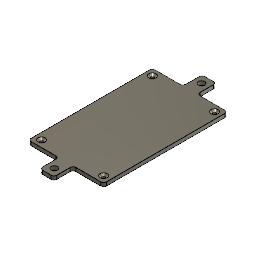
PSU Bracket v1 (Autodesk Fusion 360 design; units mm, degrees)
Autodesk Fusion 360 part; units mm, degrees
sketch "Sketch1" plane through (0, 0, 0) normal (0, 1, 0) x (1, 0, 0)
  line L0 (32.5, 58) -> (-32.5, 58) construction
  line L1 (-32.5, 58) -> (-32.5, -58) construction
  line L2 (-32.5, -58) -> (32.5, -58) construction
  line L3 (32.5, -58) -> (32.5, 58) construction
  line L4 (32.5, 58) -> (-32.5, -58) construction
  line L5 (-32.5, 58) -> (32.5, -58) construction
  circle A0 centre (32.5, 58) radius 1.75
  line L6 (0, 0) -> (0, 14) construction
  line L7 (0, 0) -> (-15, 0) construction
  circle A1 centre (-32.5, 58) radius 1.75
  circle A2 centre (32.5, -58) radius 1.75
  circle A3 centre (-32.5, -58) radius 1.75
  line L8 (39.5, 65) -> (-39.5, 65)
  line L9 (-39.5, 65) -> (-39.5, -65)
  line L10 (-39.5, -65) -> (39.5, -65)
  line L11 (39.5, -65) -> (39.5, 65)
  line L12 (39.5, 65) -> (-39.5, -65) construction
  line L13 (-39.5, 65) -> (39.5, -65) construction
  line L14 (7.5, 85) -> (-7.5, 85)
  line L15 (-7.5, 85) -> (-7.5, 65)
  line L16 (-7.5, 65) -> (7.5, 65)
  line L17 (7.5, 65) -> (7.5, 85)
  line L18 (7.5, 85) -> (-7.5, 65) construction
  line L19 (-7.5, 85) -> (7.5, 65) construction
  circle A4 centre (0, 77) radius 3.25
  line L20 (-7.5, -85) -> (-7.5, -65)
  line L21 (7.5, -85) -> (-7.5, -85)
  line L22 (-7.5, -85) -> (7.5, -65) construction
  circle A5 centre (0, -77) radius 3.25
  line L23 (-7.5, -65) -> (7.5, -65)
  line L24 (7.5, -65) -> (7.5, -85)
  line L25 (7.5, -85) -> (-7.5, -65) construction
  point P0 (0, 75)
  point P1 (0, -75)
  dimension "d1" = 116
  dimension "d2" = 65
  dimension "d3" = 3.5
  dimension "d4" = 7
  dimension "d5" = 7
  dimension "d6" = 20
  dimension "d7" = 15
  dimension "d8" = 6.5
  dimension "d9" = 12
  constraint perpendicular L0 L1
  constraint parallel L0 L2
  constraint parallel L1 L3
  constraint horizontal L0
  constraint coincident L4 L6.start
  constraint coincident L5 L6.start
  constraint coincident L6.start L7.start
  constraint coincident L0.start L3.end
  constraint vertical L6
  constraint perpendicular L6 L7
  constraint symmetric A0 L6 A1
  constraint symmetric A0 L7 A2
  constraint symmetric L7 A1 A3
  constraint perpendicular L8 L9
  constraint parallel L8 L10
  constraint parallel L9 L11
  constraint horizontal L8
  constraint coincident L12 L6.start
  constraint coincident L13 L6.start
  constraint perpendicular L14 L15
  constraint parallel L14 L16
  constraint parallel L15 L17
  constraint horizontal L14
  constraint coincident L18 P0
  constraint coincident L19 P0
  constraint collinear L8 L16
  constraint coincident L6 P0
  constraint coincident L6 A4.centre
  constraint symmetric L7 L14.start L21.start
  constraint symmetric L7 L14.end L20.start
  constraint symmetric L7 L15.end L20.end
  constraint symmetric L7 L16.end L22.end
  constraint symmetric L7 P0 P1
  constraint symmetric L7 A4 A5
  measures "d1" distance of L0.start L2.end
  measures "d2" distance of L0.start L0.end
  measures "d3" diameter of A0
  measures "d4" distance of L0.start L8
  measures "d5" distance of L0.start L11
  measures "d6" distance of L14 L16
  measures "d7" distance of L15 L17
  measures "d8" diameter of A4
  measures "d9" distance of L8 A4.centre
extrude "Extrude1" add sketch "Sketch1" along normal blind 4
fillet "Fillet1" radius 3 12 edges at (-39.5, 2, 65) (-7.5, 2, 85) (7.5, 2, 85) (7.5, 2, 65) (39.5, 2, 65) (39.5, 2, -65) (7.5, 2, -65) (7.5, 2, -85) (-7.5, 2, -85) (-39.5, 2, -65) (-7.5, 2, -65) (-7.5, 2, 65)
chamfer "Chamfer2" distance 2 angle 45 4 edges at (-34.1316, 4, 57.3672) (30.8684, 4, 57.3672) (30.8684, 4, -58.6328) (-34.1316, 4, -58.6328)
